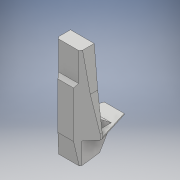
# Autodesk Inventor part: newbody
Saved by Autodesk Inventor 2018.1 (Build 221171000, 171)
## iProperties
Created: 2017-10-10
Part Number: newbody
Material: 一般
Document SubType Name: Modeling
Designer: kuwano
Density: 1 g/cm^3
Appearance: 既定
Author: kuwano
Autodesk Inventor part; units mm, degrees
ref_plane "YZ Plane" through (0, 0, 0) normal (1, 0, 0) x (0, 1, 0)
ref_plane "XZ Plane" through (0, 0, 0) normal (0, 1, 0) x (-1, 0, 0)
ref_plane "XY Plane" through (0, 0, 0) normal (0, 0, 1) x (1, 0, 0)
sketch "スケッチ1" plane through (0, 0, 0) normal (0, 0, 1) x (1, 0, 0)
  line L0 (-341.5, 417.85) -> (341.5, 417.85)
  line L1 (341.5, 417.85) -> (341.5, -417.85)
  line L2 (341.5, -417.85) -> (-341.5, -417.85)
  line L3 (-341.5, -417.85) -> (-341.5, 417.85)
  line L4 (-478.1, 0) -> (478.1, 0) projected
  line L5 (0, -584.99) -> (0, 584.99) projected
  point P0 (0, 0)
  point P1 (341.5, 0)
  point P2 (0, 417.85)
  dimension "d2" = 835.7
  dimension "d3" = 683
  constraints: 8 end point, 2 midpoint, 2 parallel, 2 point on line, 1 horizontal, 1 perpendicular
  measures "d2" distance of L0.end L1.end
  measures "d3" distance of L0.start L0.end
extrude "押し出し1" add sketch "スケッチ1" along normal blind 1357
sketch "スケッチ3" plane through (0, 0, 0) normal (0, 0, 1) x (1, 0, 0)
  line L0 (-171.5, 417.85) -> (171.5, 417.85)
  line L1 (171.5, 417.85) -> (341.5, -132.15)
  line L2 (341.5, -132.15) -> (341.5, -166.8)
  line L3 (341.5, -166.8) -> (135, -417.85)
  line L4 (-341.5, 417.85) -> (341.5, 417.85) projected
  line L5 (341.5, 417.85) -> (341.5, -417.85) projected
  line L6 (341.5, -417.85) -> (-341.5, -417.85) projected
  line L7 (0, -595.6665) -> (0, 649.0488) projected
  line L8 (135, -417.85) -> (0, -417.85)
  line L9 (-341.5, -417.85) -> (341.5, -417.85) projected
  line L10 (-171.5, 417.85) -> (-341.5, -132.15)
  line L11 (-341.5, -132.15) -> (-341.5, -166.8)
  line L12 (-341.5, -166.8) -> (-135, -417.85)
  line L13 (-135, -417.85) -> (0, -417.85)
  line L14 (341.5, 417.85) -> (-341.5, 417.85) projected
  line L15 (171.5, 417.85) -> (341.5, 417.85)
  line L16 (341.5, 417.85) -> (341.5, -132.15)
  line L17 (341.5, -417.85) -> (341.5, 417.85) projected
  line L18 (341.5, -166.8) -> (341.5, -417.85)
  line L19 (341.5, -417.85) -> (135, -417.85)
  line L20 (-135, -417.85) -> (-341.5, -417.85)
  line L21 (-341.5, -417.85) -> (-341.5, -166.8)
  line L22 (-341.5, 417.85) -> (-341.5, -417.85) projected
  line L23 (-171.5, 417.85) -> (-341.5, 417.85)
  line L24 (-341.5, -132.15) -> (-341.5, 417.85)
  point P0 (0, 0)
  point P1 (0, 417.85)
  dimension "d9" = 343
  dimension "d10" = 34.65
  dimension "d11" = 550
  dimension "d12" = 206.5
  constraints: 34 end point, 9 collinear, 3 symmetric about line, 2 midpoint, 2 perpendicular, 2 point on line, 1 horizontal
  measures "d9" distance of L0.start L0.end
  measures "d10" distance of L1.end L2.end
  measures "d11" distance from line of L1.end L4
  measures "d12" distance from line of L3.end L5
extrude "押し出し2" cut sketch "スケッチ3" along normal through all both and the other way through all contours L10 L22 L4 | L4 L5 L1 | L12 L6 L21 | L3 L5 L6
sketch "スケッチ5" plane through (0, 0, 1357) normal (0, 0, 1) x (1, 0, 0)
  line L0 (-171.5, 417.85) -> (-341.5, -132.15) projected
  line L1 (-341.5, -132.15) -> (-171.5, 417.85)
  line L2 (171.5, 417.85) -> (-171.5, 417.85) projected
  line L3 (-171.5, 417.85) -> (171.5, 417.85)
  line L4 (341.5, -132.15) -> (171.5, 417.85) projected
  line L5 (171.5, 417.85) -> (341.5, -132.15)
  line L6 (341.5, -132.15) -> (-341.5, -132.15)
  point P0 (0, 0)
  constraints: 8 end point, 3 collinear, 1 parallel
extrude "押し出し3" cut sketch "スケッチ5" against normal blind 1337
sketch "スケッチ6" plane through (-341.5, -132.15, 1357) normal (0, 1, 0) x (1, 0, 0)
  line L0 (0, 1265.7) -> (0, 665.7)
  line L1 (0, 665.7) -> (76.7, 665.7)
  line L2 (76.7, 665.7) -> (0, 1265.7)
  line L3 (0, 1357) -> (170, 1357) projected
  line L4 (0, 0) -> (0, 1337) projected
  line L5 (341.5, 1357) -> (341.5, 1610.7019)
  line L6 (683, 1265.7) -> (683, 665.7)
  line L7 (683, 665.7) -> (606.3, 665.7)
  line L8 (606.3, 665.7) -> (683, 1265.7)
  line L9 (0, 665.7) -> (76.7, 665.7)
  line L10 (0, 665.7) -> (0, 0)
  line L11 (0, 1357) -> (0, 0) projected
  line L12 (76.7, 665.7) -> (136.7, 0)
  line L13 (206.5, 0) -> (206.5, 1357) projected
  line L14 (0, 0) -> (136.7, 0)
  line L15 (683, 0) -> (0, 0) projected
  line L16 (683, 665.7) -> (606.3, 665.7)
  line L17 (683, 665.7) -> (606.3, 665.7)
  line L18 (683, 665.7) -> (683, 0)
  line L19 (606.3, 665.7) -> (546.3, 0)
  line L20 (683, 0) -> (546.3, 0)
  point P0 (683, 0)
  dimension "d17" = 91.3
  dimension "d18" = 600
  dimension "d19" = 76.7
  dimension "d21" = 60
  constraints: 32 end point, 6 symmetric about line, 3 collinear, 2 perpendicular, 2 vertical, 1 point on line
  measures "d17" distance from line of L0.start L3
  measures "d18" distance of L0.start L0.end
  measures "d19" distance of L0.end L1.end
  measures "d21" horizontal distance of L12.end L1.end
extrude "押し出し4" cut sketch "スケッチ6" against normal through all
sketch "スケッチ7" plane through (0, 0, 0) normal (1, 0, 0) x (0, 1, 0)
  line L0 (-332.9915, 1357) -> (-417.85, 1357) projected
  line L1 (-371.05, 1357) -> (-417.85, 1357)
  line L2 (-417.85, 1357) -> (-417.85, 799.8485)
  line L3 (-417.85, 1357) -> (-417.85, 0) projected
  line L4 (-417.85, 799.8485) -> (-371.05, 862.4972)
  line L5 (-371.05, 862.4972) -> (-371.05, 1357)
  line L6 (-332.9915, 1357) -> (-260.0471, 691.3) projected
  line L7 (-417.85, 0) -> (-417.85, 1357) projected
  point P0 (0, 0)
  dimension "d25" = 143.239
  dimension "d26" = 46.8
  constraints: 8 end point, 2 point on line, 1 collinear, 1 parallel
  measures "d25" angle of L3 L4
  measures "d26" distance between parallel lines of L2 L5
extrude "押し出し5" cut sketch "スケッチ7" along normal through all both and the other way through all
sketch "スケッチ8" plane through (0, 0, 0) normal (1, 0, 0) x (0, 1, 0)
  line L0 (-132.15, 20) -> (417.85, 20) projected
  line L1 (167.85, 20) -> (-132.15, 252.8315)
  line L2 (-132.15, 91.3) -> (-132.15, 691.3) projected
  line L3 (-132.15, 20) -> (-132.15, 91.3) projected
  line L4 (-132.15, 252.8315) -> (-132.15, 20)
  line L5 (-132.15, 20) -> (167.85, 20)
  point P0 (0, 0)
  dimension "d29" = 37.815
  dimension "d30" = 300
  constraints: 6 end point, 2 point on line, 1 collinear, 1 perpendicular
  measures "d29" angle of L0 L1
  measures "d30" distance of L0.start L1.start
extrude "押し出し6" add sketch "スケッチ8" along normal mid plane 400
sketch "スケッチ9" plane through (0, 0, 0) normal (1, 0, 0) x (0, 1, 0)
  line L0 (159.383, 0) -> (-34.9495, -326.55)
  line L1 (-34.9495, -326.55) -> (-365.0355, -370.5068)
  line L2 (-365.0355, -370.5068) -> (-417.85, 0)
  line L3 (-772.2018, 0) -> (616.192, 0) projected
  line L4 (-417.85, 0) -> (-417.85, 799.8485) projected
  point P0 (0, 0)
  dimension "d33" = 171.887
  dimension "d34" = 128.343
  dimension "d35" = 90.527
  dimension "d36" = 380
  dimension "d37" = 333
  constraints: 6 end point, 1 point on line
  measures "d33" angle of L4 L2
  measures "d34" angle of L0 L1
  measures "d35" angle of L2 L1
  measures "d36" distance of L0.start L0.end
  measures "d37" distance of L0.end L1.end
extrude "押し出し7" add sketch "スケッチ9" along normal mid plane 400
sketch "スケッチ10" plane through (0, 0, 0) normal (0, 0, 1) x (1, 0, 0)
  line L0 (-200, -338.827) -> (-341.5, -166.8) projected
  line L1 (-200, -365.0355) -> (-200, -417.85) projected
  line L2 (-200, -338.827) -> (-200, -417.85)
  line L3 (-135, -417.85) -> (-200, -417.85) projected
  line L4 (-200, -417.85) -> (-135, -417.85)
  line L5 (-135, -417.85) -> (-200, -338.827)
  line L6 (200, -338.827) -> (200, 159.383) projected
  line L7 (200, -338.827) -> (135, -417.85) projected
  line L8 (200, -338.827) -> (135, -417.85)
  line L9 (200, -417.85) -> (135, -417.85) projected
  line L10 (135, -417.85) -> (200, -417.85)
  line L11 (200, -417.85) -> (200, -338.827)
  point P0 (0, 0)
  constraints: 12 end point, 3 collinear, 1 perpendicular, 1 vertical
extrude "押し出し8" cut sketch "スケッチ10" against normal through all
